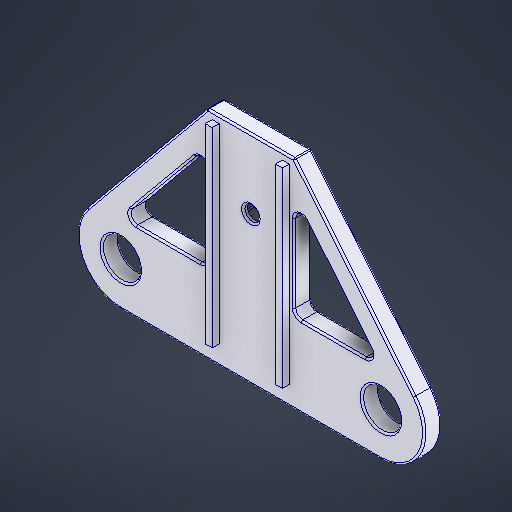
# Autodesk Inventor part: BandeV2Base
Saved by Autodesk Inventor 2026.3 (Build 303398000, 398)
## iProperties
Created: 2026-06-25
Part Number: BandeV2Base
Material: PET Plastic
Document SubType Name: Modeling
Designer: frede
Density: 1.541 g/cm^3
Appearance: Cool White
Author: frede
Autodesk Inventor part; units mm, degrees
ref_plane "YZ Plane" through (0, 0, 0) normal (1, 0, 0) x (0, 1, 0)
ref_plane "XZ Plane" through (0, 0, 0) normal (0, 1, 0) x (-1, 0, 0)
ref_plane "XY Plane" through (0, 0, 0) normal (0, 0, 1) x (1, 0, 0)
sketch "Sketch2" plane through (0, 0, 0) normal (0, 0, 1) x (1, 0, 0)
  circle A0 centre (0, 0) radius 5.5
  circle A1 centre (75, 0) radius 5.5
  arc A2 (-9.6472, 7.9486) -> (0, -12.5) centre (0, 0) ccw
  arc A3 (75, -12.5) -> (84.6472, 7.9486) centre (75, 0) ccw
  line L0 (0, -12.5) -> (75, -12.5)
  line L1 (50, 50) -> (25, 50)
  line L2 (25, 50) -> (-9.6472, 7.9486)
  line L3 (50, 50) -> (84.6472, 7.9486)
  line L4 (70.4827, 10.5593) -> (52, 10.5593)
  line L5 (50, 12.5593) -> (50, 34.9918)
  line L6 (53.5436, 36.2636) -> (72.0263, 13.8311)
  line L7 (37.5, 50) -> (37.5, -12.5)
  arc A4 (53.5436, 36.2636) -> (50, 34.9918) centre (52, 34.9918) ccw
  arc A5 (70.4827, 10.5593) -> (72.0263, 13.8311) centre (70.4827, 12.5593) ccw
  arc A6 (50, 12.5593) -> (52, 10.5593) centre (52, 12.5593) ccw
  line L8 (4.5173, 10.5593) -> (23, 10.5593)
  line L9 (25, 12.5593) -> (25, 34.9918)
  line L10 (21.4564, 36.2636) -> (2.9737, 13.8311)
  arc A7 (25, 34.9918) -> (21.4564, 36.2636) centre (23, 34.9918) ccw
  arc A8 (2.9737, 13.8311) -> (4.5173, 10.5593) centre (4.5173, 12.5593) ccw
  arc A9 (23, 10.5593) -> (25, 12.5593) centre (23, 12.5593) ccw
  circle A10 centre (37.5, 30) radius 2.2
  point P0 (50, 40.5644)
  point P1 (74.722, 10.5593)
  point P2 (50, 10.5593)
  dimension "d1" = 11
  dimension "d2" = 11
  dimension "d3" = 25
  dimension "d4" = 25
  dimension "d6" = 75
  dimension "d8" = 50
  dimension "d10" = 25
  dimension "d12" = 25
  dimension "d13" = 25
  dimension "d15" = 6
  dimension "d18" = 2
  dimension "d19" = 4.4
  dimension "d32" = 20
  constraints: 22 end point, 16 point on circle, 11 centre point, 9 symmetric about line, 9 tangent, 6 point on line, 3 coincident, 3 parallel, 2 equal radius, 2 midpoint, 1 perpendicular, 1 vertical, 3 other
  measures "d1" diameter of A0
  measures "d2" diameter of A1
  measures "d3" diameter of A2
  measures "d4" diameter of A3
  measures "d6" distance of A3.centre A2.centre
  measures "d8" distance from line of point (0, 0) L1
  measures "d10" distance of L1.start L1.end
  measures "d12" horizontal distance of L1.end point (0, 0)
  measures "d13" distance from line of A1.centre L5
  measures "d15" distance between parallel lines of L3 L6
  measures "d18" radius of A4
  measures "d19" diameter of A10
  measures "d32" distance from line of L1 A10.centre
extrude "Extrusion1" add sketch "Sketch2" along normal blind 5 contours L2 L1 L7 A10 L0 A2 | L7 A10 L1 L3 A3 L0
sketch "Sketch3" plane through (0, 0, 0) normal (0, 0, -1) x (-1, 0, 0)
  circle A0 centre (-37.5, 30) radius 2.2 projected
  line L0 (-33.9, 27.9215) -> (-37.5, 25.8431)
  line L1 (-37.5, 25.8431) -> (-41.1, 27.9215)
  line L2 (-41.1, 27.9215) -> (-41.1, 32.0785)
  line L3 (-41.1, 32.0785) -> (-37.5, 34.1569)
  line L4 (-37.5, 34.1569) -> (-33.9, 32.0785)
  line L5 (-33.9, 32.0785) -> (-33.9, 27.9215)
  point P0 (0, 0)
  dimension "d20" = 7.2
  constraints: 12 end point, 1 coincident, 13 other
  measures "d20" distance between parallel lines of L5 L2
extrude "Extrusion2" cut sketch "Sketch3" against normal blind 3.25
fillet "Fillet1" radius 0.5 57 edges at (33.9, 30, 0) (35.7, 33.1177, 0) (39.3, 33.1177, 0) (41.1, 30, 0) (39.3, 26.8823, 0) (35.7, 26.8823, 0) (24.4142, 11.1451, 0) (13.7586, 10.5593, 0) (2.7084, 11.7059, 0) (12.2151, 25.0473, 0) (23.6756, 36.8742, 0) (25, 23.7755, 0) (51.3244, 36.8742, 0) (62.7849, 25.0473, 0) (72.2916, 11.7059, 0) (61.2414, 10.5593, 0) (50.5858, 11.1451, 0) (50, 23.7755, 0) (86.305, -5.3335, 0) (37.5, -12.5, 0) (-11.305, -5.3335, 0) (7.6764, 28.9743, 0) (67.3236, 28.9743, 0) (37.5, 50, 0) (37.5, 50, 5) (86.305, -5.3335, 5) (37.5, -12.5, 5) (-11.305, -5.3335, 5) (7.6764, 28.9743, 5) (67.3236, 28.9743, 5) (23.6756, 36.8742, 5) (25, 23.7755, 5) (24.4142, 11.1451, 5) (13.7586, 10.5593, 5) (2.7084, 11.7059, 5) (12.2151, 25.0473, 5) (72.2916, 11.7059, 5) (61.2414, 10.5593, 5) (50.5858, 11.1451, 5) (50, 23.7755, 5) (51.3244, 36.8742, 5) (62.7849, 25.0473, 5) (-5.5, 0, 0) (-5.5, 0, 5) (69.5, 0, 0) (69.5, 0, 5) (35.3, 30, 3.25) (35.3, 30, 5) (33.9, 30, 3.25) (35.7, 33.1177, 3.25) (39.3, 33.1177, 3.25) (41.1, 30, 3.25) (39.3, 26.8823, 3.25) (35.7, 26.8823, 3.25) (33.9, 27.9215, 1.625) (25, 50, 2.5) (50, 50, 2.5)
sketch "Sketch4" plane through (0, 0, 5) normal (0, 0, 1) x (1, 0, 0)
  line L0 (26.4, -7) -> (28.4, -7)
  line L1 (28.4, -7) -> (28.4, 48)
  line L2 (28.4, 48) -> (26.4, 48)
  line L3 (26.4, 48) -> (26.4, -7)
  line L4 (46.6, -7) -> (48.6, -7)
  line L5 (48.6, -7) -> (48.6, 48)
  line L6 (48.6, 48) -> (46.6, 48)
  line L7 (46.6, 48) -> (46.6, -7)
  circle A0 centre (37.5, 30) radius 2.7 projected
  line L8 (49.7641, 50) -> (25.2359, 50) projected
  point P0 (0, 0)
  dimension "d24" = 9.1
  dimension "d25" = 18.2
  dimension "d26" = 2
  dimension "d27" = 2
  dimension "d30" = 55
  dimension "d31" = 2
  constraints: 16 end point, 4 parallel, 2 horizontal, 2 perpendicular, 2 point on line
  measures "d24" distance from line of L1 A0.centre
  measures "d25" distance between parallel lines of L7 L1
  measures "d26" distance between parallel lines of L5 L7
  measures "d27" distance between parallel lines of L1 L3
  measures "d30" distance between parallel lines of L4 L6
  measures "d31" distance between parallel lines of L8 L6
extrude "Extrusion3" add sketch "Sketch4" along normal blind 2 contours L3 L2 L1 L0 | L7 L6 L5 L4
equation "\"d12\" = -0.5 * d10 + 0.5 * d6"
equation "\"d13\" = d12"
equation "\"d24\" = 0.5 * d25"
equation "\"d27\" = d26"
body "Solid1"
